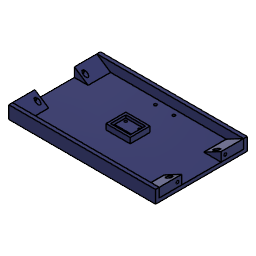
Abajo 1 (Autodesk Fusion 360 design; units mm, degrees)
Autodesk Fusion 360 part; units mm, degrees
note: some values were not read from the file. Chosen so that the rebuilt part matches the saved one: which bodies a step acts on; which face or edge a step refers to. Set by a fixed rule: which sketch regions a step uses.
sketch "Boceto1" plane through (0, 0, 0) normal (0, 1, 0) x (1, 0, 0)
  line L0 (-50, 25) -> (110, 25)
  line L1 (110, 25) -> (110, -75)
  line L2 (110, -75) -> (-50, -75)
  line L3 (-50, -75) -> (-50, 25)
  dimension "d1" = 160
  dimension "d2" = 100
  constraint horizontal L0
  constraint perpendicular L0 L1
  constraint perpendicular L1 L2
  constraint perpendicular L0 L3
  measures "d1" distance of L0.start L0.end
  measures "d2" distance of L0.end L1.end
extrude "Extruir1" add sketch "Boceto1" along normal blind 4 makes body 1
sketch "Boceto2" plane through (0, 4, 0) normal (0, 1, 0) x (-1, 0, 0)
  line L0 (50, 75) -> (-110, 75)
  line L1 (-110, 75) -> (-110, -25)
  line L2 (-110, -25) -> (50, -25)
  line L3 (50, -25) -> (50, 75)
  line L4 (50, -25) -> (50, -21)
  line L5 (50, -21) -> (-110, -21)
  line L6 (-110, -25) -> (50, -25)
  line L7 (50, 75) -> (50, 71)
  line L8 (-110, 75) -> (50, 75)
  line L9 (-110, 75) -> (-110, 71)
  line L10 (50, 71) -> (-110, 71)
  dimension "d5" = 4
  dimension "d6" = 4
  dimension "d14" = 4
  constraint coincident L2.end L3.start
  constraint perpendicular L2 L4
  constraint coincident L1 L5.end
  constraint perpendicular L1 L5
  constraint coincident L1.end L2.start
  constraint coincident L0.start L3.end
  constraint perpendicular L0 L7
  constraint coincident L0.end L1.start
  constraint perpendicular L8 L9
  measures "d5" distance of L2.end L4.end
  measures "d6" distance of L0.start L7.end
  measures "d14" distance of L0.end L9.end
extrude "Extruir2" add sketch "Boceto2" along normal blind 10 contours L0 L1 L3 L7 L8 L9 L10 | L1 L2 L3 L4 L5 L6 bodies 1
sketch "Boceto3" plane through (0, 4, 0) normal (0, 1, 0) x (-1, 0, 0)
  line L0 (-110, 71) -> (-110, -21)
  line L1 (-110, -21) -> (50, -21)
  line L2 (50, -21) -> (50, 71)
  line L3 (50, 71) -> (-110, 71)
sketch "Boceto4" plane through (0, 0, -21) normal (0, 0, 1) x (1, 0, 0)
  line L0 (-50, 4) -> (110, 4)
  line L1 (110, 4) -> (110, 14)
  line L2 (110, 14) -> (-50, 14)
  line L3 (-50, 14) -> (-50, 4)
  line L4 (-50, 0) -> (-50, 4)
  line L5 (-50, 4) -> (-50, 14)
  line L6 (-50, 4) -> (-35, 4)
  line L7 (-50, 14) -> (-35, 4)
  line L8 (110, 4) -> (91, 4)
  line L9 (110, 4) -> (110, 14)
  line L10 (110, 14) -> (91, 4)
  dimension "d9" = 10
  dimension "d10" = 19
  dimension "d11" = 10
  constraint coincident L0.start L3.end
  constraint perpendicular L0 L4
  constraint perpendicular L2 L5
  constraint coincident L0 L6.end
  constraint coincident L0.end L1.start
  constraint perpendicular L1 L8
  constraint perpendicular L0 L9
  measures "d9" distance of L0.start L2.end
  measures "d10" distance of L0.end L8.end
  measures "d11" distance of L0.end L1.end
extrude "Extruir3" add sketch "Boceto4" along normal blind 92 separate body contours L0 L3 L5 L6 L7 | L0 L1 L8 L9 L10 makes body 2 at (-45, 10.6667, 9.6667) makes body 3 at (103.6667, 10.6667, 9.6667)
sketch "Boceto6" plane through (0, 0, 71) normal (0, 0, -1) x (-1, 0, 0)
  line L0 (-110, 4) -> (50, 4)
  line L1 (50, 4) -> (50, 14)
  line L2 (50, 14) -> (-110, 14)
  line L3 (-110, 14) -> (-110, 4)
  line L4 (-110, 4) -> (-106, 4)
  line L5 (-106, 4) -> (-106, 9)
  line L6 (-110, 4) -> (-106, 4)
  line L7 (-106, 4) -> (-91, 4)
  line L8 (-91, 4) -> (-91, 9)
  line L9 (-91, 4) -> (-91, 9)
  dimension "d15" = 5
  constraint coincident L0.start L3.end
  constraint coincident L0 L4.end
  constraint perpendicular L0 L5
  constraint coincident L0 L7.end
  constraint perpendicular L7 L8
  measures "d15" distance of L4.end L5.end
sketch "Boceto7" plane through (0, 0, 0) normal (1, 0, 0) x (0, 0, -1)
  line L0 (-71, 4) -> (-71, 9)
  line L1 (-71, 9) -> (-69, 9)
  line L2 (-69, 9) -> (-51, 9)
  circle A0 centre (-51, 9) radius 2
  line L3 (-51, 9) -> (1, 9)
  circle A1 centre (1, 9) radius 2
  dimension "d16" = 2
  dimension "d17" = 18
  dimension "d22" = 4
  dimension "d31" = 52
  dimension "d32" = 4
  constraint vertical L0
  constraint perpendicular L0 L1
  constraint perpendicular L0 L2
  constraint coincident L2.end A0.centre
  constraint parallel L2 L3
  constraint coincident L3.end A1.centre
  measures "d16" distance of L0.end L1.end
  measures "d17" distance of L1.end L2.end
  measures "d22" diameter of A0
  measures "d31" distance of L2.end L3.end
  measures "d32" diameter of A1
extrude "Extruir4" cut sketch "Boceto7" along normal blind 104 contours L2 A0 L3 | L2 A0 L3 bodies 3
extrude "Extruir5" cut sketch "Boceto7" against normal blind 45.5 contours L2 A0 L3 | L2 A0 L3 bodies 2
sketch "Boceto9" plane through (-50, 0, 0) normal (-1, 0, 0) x (0, 0, 1)
  line L0 (-25, 0) -> (75, 0)
  line L1 (75, 0) -> (75, 14)
  line L2 (75, 14) -> (71, 14)
  line L3 (71, 14) -> (71, 4)
  line L4 (71, 4) -> (-21, 4)
  line L5 (-21, 4) -> (-21, 14)
  line L6 (-21, 14) -> (-25, 14)
  line L7 (-25, 14) -> (-25, 0)
  circle A0 centre (-1, 9) radius 1.5
  circle A1 centre (51, 9) radius 1.5
  dimension "d25" = 3
  dimension "d26" = 3
  measures "d25" diameter of A0
  measures "d26" diameter of A1
extrude "Extruir6" cut sketch "Boceto9" along normal mid plane 394 contours A0 | A1 bodies 3
extrude "Extruir8" cut sketch "Boceto7" against normal blind 45.5 contours A1 bodies 2
extrude "Extruir9" cut sketch "Boceto7" along normal blind 104 contours A1 bodies 3
extrude "Extruir7" cut sketch "Boceto9" against normal blind 56 contours A0 | A1 bodies 2
sketch "Boceto10" plane through (110, 0, 0) normal (1, 0, 0) x (0, 0, -1)
  circle A0 centre (1, 9) radius 1.5
  circle A1 centre (-51, 9) radius 1.5
  line L0 (21, 4) -> (21, 14)
  line L1 (21, 14) -> (-71, 14)
  line L2 (-71, 14) -> (-71, 4)
  line L3 (-71, 4) -> (21, 4)
  line L4 (-51, 9) -> (-51, 14)
  line L5 (-25, 14) -> (-3.5, 14)
  line L6 (-3.5, 14) -> (-3.5, 4)
  line L7 (-3.5, 4) -> (-46.5, 4)
  line L8 (-46.5, 4) -> (-46.5, 14)
  line L9 (-25, 14) -> (-46.5, 14)
  dimension "d37" = 21.5
  dimension "d38" = 43
  constraint coincident A1.centre L4.start
  constraint coincident L1 L4.end
  constraint perpendicular L1 L4
  constraint midpoint L1 L5.start
  constraint coincident L1 L5.end
  constraint coincident L3 L6.end
  constraint perpendicular L3 L6
  constraint perpendicular L6 L7
  constraint coincident L1 L8.end
  constraint perpendicular L1 L8
  measures "d37" distance of L5.start L5.end
  measures "d38" distance of L6.end L7.end
extrude "Extruir10" cut sketch "Boceto10" against normal blind 209 contours L1 L3 L5 L6 L7 L8 L9 bodies 2 3 makes body 5 at (100.5, 9, -15) makes body 4 at (-42.5, 9, -15)
sketch "Boceto11" plane through (0, 4, 0) normal (0, 1, 0) x (-1, 0, 0)
  line L0 (50, 71) -> (-110, 71)
  line L1 (-110, 71) -> (-110, -21)
  line L2 (-110, -21) -> (50, -21)
  line L3 (50, -21) -> (50, 71)
  line L4 (50, -25) -> (-30, -25)
  line L5 (-30, -25) -> (-30, 25)
  dimension "d41" = 80
  dimension "d42" = 50
  constraint perpendicular L1 L4
  constraint perpendicular L2 L5
  measures "d41" distance of L4.start L4.end
  measures "d42" distance of L4.end L5.end
sketch "Boceto12" plane through (0, 4, 0) normal (0, 1, 0) x (-1, 0, 0)
sketch "Boceto13" plane through (0, 4, 0) normal (0, 1, 0) x (-1, 0, 0)
  line L0 (50, 75) -> (-30, 75)
  line L1 (-30, 75) -> (-30, 25)
  line L2 (-30, 25) -> (-40.13, 25)
  line L3 (-40.13, 25) -> (-40.13, 17.22)
  line L4 (-40.13, 17.22) -> (-19.87, 17.22)
  line L5 (-19.87, 17.22) -> (-19.87, 32.78)
  line L6 (-19.87, 32.78) -> (-40.13, 32.78)
  line L7 (-40.13, 32.78) -> (-40.13, 25)
  line L8 (-19.87, 17.22) -> (-19.87, 14.22)
  line L9 (-19.87, 14.22) -> (-40.13, 14.22)
  line L10 (-40.13, 14.22) -> (-43.13, 14.22)
  line L11 (-43.13, 14.22) -> (-43.13, 32.78)
  line L12 (-43.13, 32.78) -> (-43.13, 35.78)
  line L13 (-43.13, 35.78) -> (-19.87, 35.78)
  line L14 (-19.87, 35.78) -> (-16.87, 35.78)
  line L15 (-16.87, 35.78) -> (-16.87, 14.22)
  line L16 (-19.87, 14.22) -> (-16.87, 14.22)
  line L17 (-19.87, 28.1077) -> (-40.13, 28.1077)
  dimension "d43" = 10.13
  dimension "d44" = 7.78
  dimension "d45" = 20.26
  dimension "d46" = 15.56
  dimension "d47" = 3
  dimension "d48" = 3
  dimension "d49" = 3
  dimension "d50" = 3
  constraint horizontal L0
  constraint perpendicular L0 L1
  constraint perpendicular L1 L2
  constraint perpendicular L2 L3
  constraint perpendicular L3 L4
  constraint perpendicular L4 L5
  constraint perpendicular L3 L6
  constraint perpendicular L2 L7
  constraint perpendicular L4 L8
  constraint perpendicular L3 L9
  constraint perpendicular L3 L10
  constraint perpendicular L6 L11
  constraint perpendicular L6 L12
  constraint perpendicular L5 L13
  constraint perpendicular L5 L14
  constraint perpendicular L9 L15
  constraint perpendicular L15 L16
  constraint coincident L5 L17.start
  constraint coincident L7 L17.end
  constraint perpendicular L7 L17
  measures "d43" distance of L1.end L2.end
  measures "d44" distance of L2.end L3.end
  measures "d45" distance of L3.end L4.end
  measures "d46" distance of L4.end L5.end
  measures "d47" distance of L4.end L8.end
  measures "d48" distance of L9.end L10.end
  measures "d49" distance of L11.end L12.end
  measures "d50" distance of L13.end L14.end
extrude "Extruir11" add sketch "Boceto13" along normal blind 6 contours L1 L5 L6 L8 L13 L14 L15 L16 | L1 L3 L4 L6 L7 L8 L9 L10 L11 L12 L13 bodies 1
sketch "Boceto14" plane through (0, 4, 0) normal (0, 1, 0) x (-1, 0, 0)
  line L0 (-30, 25) -> (-40, 25)
  line L1 (-40, 25) -> (-40, 30)
  constraint horizontal L0
  constraint perpendicular L0 L1
sketch "Boceto15" plane through (0, 4, 0) normal (0, 1, 0) x (-1, 0, 0)
  line L0 (-30, 25) -> (-30, 17.22)
  line L1 (-30, 17.22) -> (-40.13, 17.22)
  line L2 (-40.13, 17.22) -> (-40.13, 29)
  line L3 (-30, 17.22) -> (-19.87, 17.22)
  line L4 (-19.87, 17.22) -> (-19.87, 29)
  line L5 (-19.87, 29) -> (-40.13, 29)
  dimension "d53" = 7.78
  dimension "d54" = 10.13
  dimension "d55" = 10.13
  constraint vertical L0
  constraint perpendicular L0 L1
  constraint perpendicular L1 L2
  constraint perpendicular L0 L3
  constraint perpendicular L3 L4
  constraint perpendicular L2 L5
  measures "d53" distance of L0.start L0.end
  measures "d54" distance of L0.end L1.end
  measures "d55" distance of L0.end L3.end
extrude "Extruir12" add sketch "Boceto15" along normal blind 3 bodies 1
sketch "Boceto16" plane through (0, 4, 0) normal (0, 1, 0) x (-1, 0, 0)
  circle A0 centre (-22.4149, 19.8561) radius 1.4324
  circle A1 centre (-37.4758, 19.879) radius 1.5084
sketch "Boceto17" plane through (0, 4, 0) normal (0, 1, 0) x (-1, 0, 0)
  circle A0 centre (-37.4758, 19.879) radius 1.5084
  circle A1 centre (-22.4149, 19.8561) radius 1.4324
sketch "Boceto18" plane through (0, 7, 0) normal (0, 1, 0) x (-1, 0, 0)
  line L0 (-40.13, 17.22) -> (-19.87, 17.22)
  line L1 (-19.87, 17.22) -> (-19.87, 29)
  line L2 (-19.87, 29) -> (-40.13, 29)
  line L3 (-40.13, 29) -> (-40.13, 17.22)
  circle A0 centre (-22.4149, 19.8561) radius 1.4324
  circle A1 centre (-37.4758, 19.879) radius 1.5084
extrude "Extruir13" cut sketch "Boceto18" against normal blind 44 contours A0 | A1 bodies 1
sketch "Boceto19" plane through (0, 4, 0) normal (0, 1, 0) x (-1, 0, 0)
  line L0 (-30, 25) -> (-40.13, 25)
  line L1 (-40.13, 25) -> (-40.63, 25)
  line L2 (-40.63, 25) -> (-40.63, 16.72)
  line L3 (-40.63, 16.72) -> (-19.37, 16.72)
  line L4 (-19.37, 16.72) -> (-19.37, 33.28)
  line L5 (-19.37, 33.28) -> (-40.63, 33.28)
  line L6 (-40.63, 33.28) -> (-40.63, 25)
  dimension "d62" = 10.13
  dimension "d63" = 0.5
  dimension "d64" = 8.28
  dimension "d65" = 21.26
  dimension "d66" = 16.56
  constraint horizontal L0
  constraint parallel L0 L1
  constraint perpendicular L1 L2
  constraint perpendicular L2 L3
  constraint perpendicular L3 L4
  constraint perpendicular L2 L5
  constraint perpendicular L1 L6
  measures "d62" distance of L0.start L0.end
  measures "d63" distance of L0.end L1.end
  measures "d64" distance of L1.end L2.end
  measures "d65" distance of L2.end L3.end
  measures "d66" distance of L3.end L4.end
sketch "Boceto20" plane through (0, 10, 0) normal (0, 1, 0) x (-1, 0, 0)
  line L0 (-40.13, 17.22) -> (-40.13, 32.78)
  line L1 (-40.13, 32.78) -> (-19.87, 32.78)
  line L2 (-19.87, 32.78) -> (-19.87, 17.22)
  line L3 (-19.87, 17.22) -> (-40.13, 17.22)
  line L4 (-43.13, 14.22) -> (-16.87, 14.22)
  line L5 (-16.87, 14.22) -> (-16.87, 35.78)
  line L6 (-16.87, 35.78) -> (-43.13, 35.78)
  line L7 (-43.13, 35.78) -> (-43.13, 14.22)
  line L8 (-30, 25) -> (-40.13, 25)
  line L9 (-40.13, 25) -> (-40.63, 25)
  line L10 (-40.63, 25) -> (-40.63, 17.22)
  line L11 (-40.63, 17.22) -> (-40.63, 16.72)
  line L12 (-40.63, 16.72) -> (-19.87, 16.72)
  line L13 (-19.87, 16.72) -> (-19.37, 16.72)
  line L14 (-19.37, 16.72) -> (-19.37, 32.78)
  line L15 (-19.37, 32.78) -> (-19.37, 33.28)
  line L16 (-19.37, 33.28) -> (-40.63, 33.28)
  line L17 (-40.63, 33.28) -> (-40.63, 25)
  dimension "d67" = 0.5
  dimension "d68" = 0.5
  dimension "d69" = 0.5
  dimension "d70" = 0.5
  constraint midpoint L0 L8.end
  constraint perpendicular L0 L8
  constraint perpendicular L0 L9
  constraint perpendicular L3 L10
  constraint perpendicular L3 L11
  constraint perpendicular L2 L12
  constraint perpendicular L2 L13
  constraint perpendicular L1 L14
  constraint perpendicular L1 L15
  constraint perpendicular L10 L16
  constraint perpendicular L9 L17
  measures "d67" distance of L8.end L9.end
  measures "d68" distance of L10.end L11.end
  measures "d69" distance of L12.end L13.end
  measures "d70" distance of L14.end L15.end
extrude "Extruir14" cut sketch "Boceto20" against normal blind 3 contours L10 L11 L12 L13 L14 L15 L16 L17 bodies 1
sketch "Boceto21" plane through (0, 0, 0) normal (0, -1, 0) x (1, 0, 0)
  circle A0 centre (22.4149, 19.8561) radius 1.4324
  circle A1 centre (37.4758, 19.879) radius 1.5084
  line L0 (110, 75) -> (-50, 75)
  line L1 (-50, 75) -> (-50, -25)
  line L2 (-50, -25) -> (110, -25)
  line L3 (110, -25) -> (110, 75)
  line L4 (-50, 75) -> (-15, 75)
  line L5 (-15, 75) -> (-15, 60)
  line L6 (-5, 60) -> (-5, 75)
  line L7 (-5, 75) -> (0, 75)
  line L8 (-15, 75) -> (-20, 75)
  line L9 (-20, 75) -> (-20, 45)
  line L10 (-20, 45) -> (0, 45)
  line L11 (0, 45) -> (0, 75)
  line L12 (-50, -25) -> (-20, -25)
  line L13 (-20, -25) -> (-20, 5)
  line L14 (-20, 5) -> (0, 5)
  line L15 (0, 5) -> (0, -25)
  line L16 (0, -25) -> (-5, -25)
  line L17 (-5, -25) -> (-5, 0)
  line L18 (-5, 0) -> (-15, 0)
  line L19 (-15, 0) -> (-15, -25)
  line L20 (-15, -25) -> (-20, -25)
  line L21 (110, 75) -> (80, 75)
  line L22 (80, 75) -> (80, 45)
  line L23 (80, 45) -> (60, 45)
  line L24 (60, 45) -> (60, 75)
  line L25 (60, 75) -> (65, 75)
  line L26 (65, 75) -> (65, 50)
  line L27 (65, 50) -> (75, 50)
  line L28 (75, 50) -> (75, 75)
  line L29 (110, -25) -> (80, -25)
  line L30 (80, -25) -> (80, 5)
  line L31 (80, 5) -> (61, 5)
  line L32 (61, 5) -> (61, -25)
  line L33 (61, -25) -> (63, -25)
  line L34 (80, -25) -> (75, -25)
  line L35 (75, -25) -> (75, 0)
  line L36 (75, 0) -> (65, 0)
  line L37 (65, 0) -> (65, -25)
  line L38 (-15, 60) -> (-15, 50)
  line L39 (-15, 50) -> (-5, 50)
  line L40 (-5, 50) -> (-5, 60)
  dimension "d73" = 35
  dimension "d74" = 10
  dimension "d75" = 5
  dimension "d76" = 5
  dimension "d77" = 30
  dimension "d82" = 30
  dimension "d83" = 30
  dimension "d84" = 20
  dimension "d85" = 5
  dimension "d86" = 30
  dimension "d87" = 30
  dimension "d88" = 20
  dimension "d89" = 5
  dimension "d90" = 25
  dimension "d91" = 30
  dimension "d92" = 5
  dimension "d93" = 10
  constraint coincident L0.end L1.start
  constraint perpendicular L1 L4
  constraint perpendicular L4 L5
  constraint coincident L0 L6.end
  constraint perpendicular L0 L6
  constraint perpendicular L6 L7
  constraint perpendicular L5 L8
  constraint perpendicular L4 L9
  constraint perpendicular L5 L10
  constraint perpendicular L7 L11
  constraint coincident L1.end L2.start
  constraint perpendicular L1 L12
  constraint perpendicular L12 L13
  constraint perpendicular L13 L14
  constraint coincident L2 L15.end
  constraint perpendicular L2 L15
  constraint perpendicular L15 L16
  constraint perpendicular L16 L17
  constraint perpendicular L15 L18
  constraint coincident L2 L19.end
  constraint perpendicular L2 L19
  constraint coincident L0.start L3.end
  constraint perpendicular L3 L21
  constraint perpendicular L21 L22
  constraint perpendicular L3 L23
  constraint coincident L0 L24.end
  constraint perpendicular L0 L24
  constraint coincident L0 L25.end
  constraint perpendicular L25 L26
  constraint perpendicular L26 L27
  constraint coincident L0 L28.end
  constraint perpendicular L0 L28
  constraint coincident L2.end L3.start
  constraint coincident L2 L29.end
  constraint perpendicular L29 L30
  constraint perpendicular L24 L31
  constraint coincident L2 L32.end
  constraint perpendicular L2 L32
  constraint coincident L2 L33.end
  constraint coincident L2 L34.end
  constraint perpendicular L34 L35
  constraint perpendicular L30 L36
  constraint coincident L2 L37.end
  constraint perpendicular L2 L37
  constraint perpendicular L4 L38
  constraint perpendicular L6 L39
  constraint perpendicular L39 L40
  measures "d73" distance of L0.end L4.end
  measures "d74" distance of L5.end L6.start
  measures "d75" distance of L6.end L7.end
  measures "d76" distance of L4.end L8.end
  measures "d77" distance of L8.end L9.end
  measures "d82" distance of L1.end L12.end
  measures "d83" distance of L12.end L13.end
  measures "d84" distance of L13.end L14.end
  measures "d85" distance of L15.end L16.end
  measures "d86" distance of L0.start L21.end
  measures "d87" distance of L21.end L22.end
  measures "d88" distance of L22.end L23.end
  measures "d89" distance of L24.end L25.end
  measures "d90" distance of L25.end L26.end
  measures "d91" distance of L29.end L30.end
  measures "d92" distance of L29.end L34.end
  measures "d93" distance of L5.end L38.end
sketch "Boceto22" plane through (0, -2.14, 0) normal (0, -1, 0) x (1, 0, 0)
  line L0 (-15, 75) -> (-20, 75)
  line L1 (-20, 75) -> (-20, 45)
  line L2 (-20, 45) -> (0, 45)
  line L3 (0, 45) -> (0, 75)
  line L4 (0, 75) -> (-5, 75)
  line L5 (-5, 75) -> (-5, 50)
  line L6 (-5, 50) -> (-15, 50)
  line L7 (-15, 50) -> (-15, 75)
  line L8 (-20, 75) -> (0, 75)
  line L9 (0, 75) -> (0, 45)
  line L10 (-20, 45) -> (0, 45)
  line L11 (-20, 45) -> (-20, 75)
  line L12 (60, 75) -> (80, 75)
  line L13 (80, 45) -> (60, 45)
  line L14 (60, 45) -> (60, 75)
  line L15 (80, 75) -> (80, 45)
  line L16 (-20, 5) -> (0, 5)
  line L17 (0, 5) -> (0, -25)
  line L18 (0, -25) -> (-20, -25)
  line L19 (-20, -25) -> (-20, 5)
  line L20 (61, 5) -> (80, 5)
  line L21 (80, 5) -> (80, -25)
  line L22 (80, -25) -> (61, -25)
  line L23 (61, -25) -> (61, 5)
  constraint coincident L0.end L1.start
  constraint coincident L3.end L4.start
  constraint coincident L2.end L3.start
  constraint coincident L1.end L2.start
  constraint perpendicular L1 L12
  constraint parallel L12 L13
  constraint perpendicular L12 L14
  constraint perpendicular L12 L15
  constraint horizontal L16
  constraint perpendicular L16 L17
  constraint perpendicular L17 L18
  constraint perpendicular L18 L19
  constraint perpendicular L19 L20
  constraint perpendicular L20 L21
  constraint perpendicular L21 L22
  constraint coincident L20 L23.end
  constraint perpendicular L20 L23
sketch "Boceto23" plane through (0, 4, 0) normal (0, 1, 0) x (-1, 0, 0)
  circle A0 centre (-40, 65) radius 1.5
  circle A1 centre (-20, 65) radius 1.5
  circle A2 centre (-40, -15) radius 1.5
  circle A3 centre (-20, -15) radius 1.5
extrude "Extruir17" cut sketch "Boceto23" against normal blind 25 bodies 1
equation "d43 = ( 2.026 / 2 ) * 1 cm"
equation "d44 = ( 1.556 / 2 ) * 1 cm"
equation "d53 = ( 1.556 / 2 ) * 1 cm"
equation "d54 = ( 2.026 / 2 ) * 1 cm"
equation "d62 = ( 2.026 / 2 ) * 1 cm"
equation "d64 = ( 1.556 / 2 ) * 1 cm + 0.05 cm"
equation "d65 = 2.026 cm + 0.1 cm"
equation "d66 = 1.556 cm + 0.1 cm"
